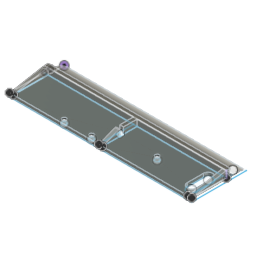
Rear-Wedge_100x30mm (Autodesk Fusion 360 design; units mm, degrees)
part number: 2026-04-11-16-21-14-908
Autodesk Fusion 360 part; units mm, degrees
sketch "Sketch1" plane through (0, 0, 0) normal (0, 0, 1) x (1, 0, 0)
  line L0 (0, 0) -> (100, 0)
  line L1 (100, 0) -> (100, -30)
  line L2 (100, -30) -> (0, -30)
  line L3 (0, -30) -> (0, 0)
  line L4 (96.5, -15) -> (96.5, -24)
  line L5 (91.5, -15) -> (91.5, -24)
  arc A0 (96.5, -15) -> (91.5, -15) centre (94, -15) ccw
  arc A1 (91.5, -24) -> (96.5, -24) centre (94, -24) ccw
  circle A2 centre (70.5, -19.5) radius 1.15
  circle A3 centre (42.5, -27.5) radius 1.15
  circle A4 centre (27.5, -27.5) radius 1.15
  dimension "d22" = 2.3
  constraint horizontal L0
  constraint vertical L1
  constraint horizontal L2
  constraint vertical L3
  constraint coincident L0.start L3.end
  constraint tangent L4 A1
  constraint vertical L4
  constraint tangent L5 A1
  constraint parallel L4 L5
  measures "d22" diameter of A2
extrude "Extrude2" add sketch "Sketch1" along normal blind 2
fillet "Fillet1" radius 15 1 edges at (50, 0, 2)
fillet "Fillet2" radius 2 2 edges at (100, -15, 0) (0, -15, 0)
sketch "Sketch2" plane through (0, 0, 2) normal (0, 0, 1) x (-1, 0, 0)
  line L0 (-100, 7.4833) -> (0, 7.4833)
  line L1 (0, 7.4833) -> (0, 30)
  line L2 (0, 30) -> (-100, 30)
  line L3 (-100, 30) -> (-100, 7.4833)
  arc A0 (-96.5, 15) -> (-91.5, 15) centre (-94, 15) ccw
  line L4 (-96.5, 15) -> (-96.5, 24)
  arc A1 (-91.5, 24) -> (-96.5, 24) centre (-94, 24) ccw
  line L5 (-91.5, 24) -> (-91.5, 15)
  circle A2 centre (-42.5, 27.5) radius 1.15
  circle A3 centre (-70.5, 19.5) radius 1.15
  circle A4 centre (-27.5, 27.5) radius 1.15
  line L6 (0, 7.4833) -> (-100, 7.4833)
  line L7 (0, 11) -> (-100, 11)
  line L8 (-100, 11) -> (-100, 7.4833)
  line L9 (0, 11) -> (0, 7.4833)
  line L10 (-98, 11) -> (-98, 30)
  line L11 (-2, 11) -> (-2, 30)
  line L12 (0, 11) -> (0, 30)
  line L13 (-2, 30) -> (0, 30)
  line L14 (-98, 30) -> (-100, 30)
  line L15 (-100, 11) -> (-100, 30)
  line L16 (-51, 11) -> (-51, 30)
  line L17 (-51, 30) -> (-49, 30)
  line L18 (-49, 30) -> (-49, 11)
  line L19 (-49, 20.5) -> (-51, 20.5)
  line L20 (-51, 20.5) -> (-51, 18.5)
  line L21 (-51, 18.5) -> (-49, 18.5)
  line L22 (-49, 18.5) -> (-49, 20.5)
  point P0 (-50, 19.5)
  constraint horizontal L6
  constraint coincident L0.end L1.start
  constraint coincident L1 L7.start
  constraint coincident L3 L7.end
  constraint perpendicular L3 L7
  constraint coincident L7 L10.start
  constraint coincident L2 L10.end
  constraint perpendicular L2 L10
  constraint coincident L7 L11.start
  constraint coincident L2 L11.end
  constraint perpendicular L2 L11
  constraint coincident L1.end L2.start
  constraint coincident L2.end L3.start
  constraint coincident L7 L16.start
  constraint coincident L2 L16.end
  constraint perpendicular L2 L16
  constraint coincident L2 L17.end
  constraint coincident L7 L18.end
  constraint perpendicular L7 L18
  constraint horizontal L19
  constraint perpendicular L19 L20
  constraint parallel L19 L21
  constraint parallel L20 L22
  constraint midpoint L18 L19.start
extrude "Extrude5" add sketch "Sketch2" along normal blind 3.5 contours L0 L1 L3 L6 L7 L8 L9 | L2 L3 L7 L10 L14 L15 | L1 L2 L7 L11 L12 L13 | L7 L16 L18 L21 | L2 L16 L17 L18 L19
sketch "Sketch4" plane through (100, 0, 0) normal (1, 0, 0) x (0, 1, 0)
  line L0 (-11, 2) -> (-7.4833, 2)
  line L1 (-7.4833, 2) -> (-7.4833, 5.5)
  line L2 (-7.4833, 5.5) -> (-11, 5.5)
  line L3 (-11, 5.5) -> (-11, 2)
  point P0 (-7.4833, 4)
hole "Hole4" at (100, -7.4833, 4) direction (-1, 0, 0) diameter 4 depth 100 tip angle 180
chamfer "Chamfer1" distance 19 distance2 3.5 2 edges at (99, -30, 5.5) (1, -30, 5.5) measured on face at (49.6667, -9.5375, 5.5) measured on face at (49.6667, -9.5375, 5.5)
chamfer "Chamfer2" distance 9 distance2 3.5 1 edges at (50, -30, 5.5) measured on face at (50.3333, -26.8333, 5.5)
